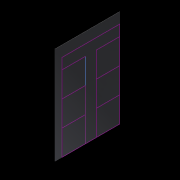
# Autodesk Inventor part: plate 1
Saved by Autodesk Inventor 2015 SP1 (Build 190203100, 203)
## iProperties
Created: 2014-10-18
Part Number: plate 1
Material: Generic
Document SubType Name: Modeling
Designer: datenney
Density: 1 g/cm^3
Appearance: Default
Author: datenney
Autodesk Inventor part; units mm, degrees
ref_plane "YZ Plane" through (0, 0, 0) normal (1, 0, 0) x (0, 1, 0)
ref_plane "XZ Plane" through (0, 0, 0) normal (0, 1, 0) x (-1, 0, 0)
ref_plane "XY Plane" through (0, 0, 0) normal (0, 0, 1) x (1, 0, 0)
sketch "Sketch1" plane through (0, 0, 0) normal (1, 0, 0) x (0, 1, 0)
  line L0 (0, 0) -> (0, -203.2)
  line L1 (0, -203.2) -> (304.8, -203.2)
  line L2 (304.8, -203.2) -> (304.8, 0)
  line L3 (304.8, 0) -> (0, 0)
  line L4 (0, 0) -> (0, -82.55)
  line L5 (0, -203.2) -> (0, -120.65)
  line L6 (0, -203.2) -> (88.9, -203.2)
  line L7 (88.9, -203.2) -> (88.9, -120.65)
  line L8 (88.9, -120.65) -> (0, -120.65)
  line L9 (0, -82.55) -> (88.9, -82.55)
  line L10 (88.9, -82.55) -> (88.9, 0)
  line L11 (88.9, 0) -> (88.9, 0)
  line L12 (88.9, 0) -> (88.9, -82.55)
  line L13 (88.9, -82.55) -> (177.8, -82.55)
  line L14 (177.8, -82.55) -> (177.8, 0)
  line L15 (88.9, -203.2) -> (88.9, -203.2)
  line L16 (88.9, -203.2) -> (88.9, -120.65)
  line L17 (177.8, -120.65) -> (177.8, -203.2)
  line L18 (88.9, -120.65) -> (177.8, -120.65)
  line L19 (177.8, -120.65) -> (266.7, -120.65)
  line L20 (266.7, -120.65) -> (266.7, -203.2)
  line L21 (177.8, -82.55) -> (266.7, -82.55)
  line L22 (266.7, -82.55) -> (266.7, 0)
  dimension "d0" = 203.2
  dimension "d1" = 304.8
  dimension "d2" = 82.55
  dimension "d3" = 82.55
  dimension "d4" = 38.1
  dimension "d5" = 88.9
  dimension "d6" = 0
  dimension "d7" = 88.9
  dimension "d8" = 88.9
  dimension "d9" = 88.9
  constraints: 46 end point, 22 point on line, 10 perpendicular, 1 parallel, 1 vertical
  measures "d0" distance of L0.start L0.end
  measures "d1" distance of L0.end L1.end
  measures "d2" distance of L0.start L4.end
  measures "d3" distance of L0.end L5.end
  measures "d4" distance of L5.end L4.end
  measures "d5" distance of L0.end L6.end
  measures "d6" distance of L10.end L11.end
  measures "d7" distance of L12.end L13.end
  measures "d8" distance of L17.start L19.end
  measures "d9" distance of L13.end L21.end
sketch "Sketch2" plane through (0, 0, 0) normal (1, 0, 0) x (0, 1, 0)
  line L0 (0, 0) -> (0, 25.4)
  line L1 (0, 25.4) -> (342.9, 25.4)
  line L2 (342.9, 25.4) -> (342.9, -203.2)
  line L3 (342.9, -203.2) -> (0, -203.2)
  line L4 (0, -203.2) -> (0, 25.4)
  dimension "d14" = 25.4
  dimension "d15" = 342.9
  dimension "d16" = 228.6
  constraints: 10 end point, 3 perpendicular, 1 collinear, 1 point on line, 1 vertical
  measures "d14" distance of L0.start L0.end
  measures "d15" distance of L0.end L1.end
  measures "d16" distance of L1.end L2.end
extrude "Extrusion1" add sketch "Sketch2" along normal blind 1.524
body "Solid1"
